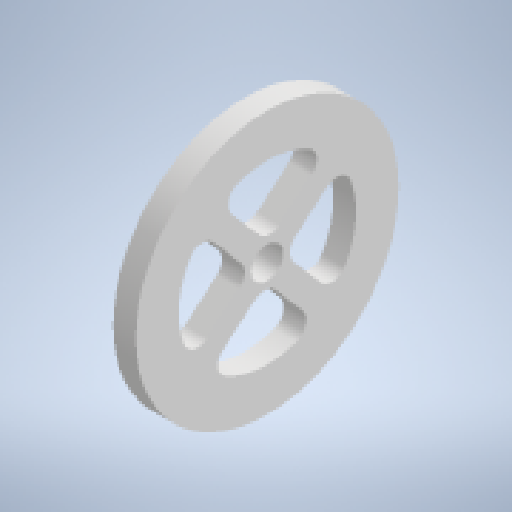
# Autodesk Inventor part: WheelBetter
Saved by Autodesk Inventor 2025.2 (Build 292293000, 293)
## iProperties
Created: 2025-02-03
Part Number: WheelBetter
Material: Generic
Document SubType Name: Modeling
Designer: andre
Density: 1 g/cm^3
Appearance: Default
Author: andre
Autodesk Inventor part; units mm, degrees
ref_plane "YZ Plane" through (0, 0, 0) normal (1, 0, 0) x (0, 1, 0)
ref_plane "XZ Plane" through (0, 0, 0) normal (0, 1, 0) x (-1, 0, 0)
ref_plane "XY Plane" through (0, 0, 0) normal (0, 0, 1) x (1, 0, 0)
sketch "Sketch1" plane through (0, 0, 0) normal (1, 0, 0) x (0, 1, 0)
  arc A0 (23.1835, 24.2674) -> (22.463, 14.9178) centre (33.5654, 18.7649) ccw
  arc A1 (26.4699, 24.6315) -> (23.1835, 24.2674) centre (24.9506, 23.3308) ccw
  line L0 (26.4699, 24.6315) -> (30.0498, 20.4497)
  arc A2 (29.8311, 17.6297) -> (30.0498, 20.4497) centre (28.5305, 19.149) ccw
  line L1 (29.8311, 17.6297) -> (25.6534, 14.0533)
  arc A3 (22.463, 14.9178) -> (25.6534, 14.0533) centre (24.3528, 15.5727) ccw
  arc A4 (28.0629, 8.3829) -> (37.4124, 7.6625) centre (33.5654, 18.7649) ccw
  arc A5 (27.6988, 11.6694) -> (28.0629, 8.3829) centre (28.9995, 10.1501) ccw
  line L2 (27.6988, 11.6694) -> (31.8806, 15.2493)
  arc A6 (34.7006, 15.0306) -> (31.8806, 15.2493) centre (33.1812, 13.73) ccw
  line L3 (34.7006, 15.0306) -> (38.277, 10.8529)
  arc A7 (37.4124, 7.6625) -> (38.277, 10.8529) centre (36.7576, 9.5523) ccw
  arc A8 (43.9473, 13.2623) -> (44.6678, 22.6119) centre (33.5654, 18.7649) ccw
  arc A9 (40.6609, 12.8983) -> (43.9473, 13.2623) centre (42.1802, 14.1989) ccw
  line L4 (40.6609, 12.8983) -> (37.081, 17.0801)
  arc A10 (37.2997, 19.9) -> (37.081, 17.0801) centre (38.6003, 18.3807) ccw
  line L5 (37.2997, 19.9) -> (41.4774, 23.4764)
  arc A11 (44.6678, 22.6119) -> (41.4774, 23.4764) centre (42.778, 21.9571) ccw
  line L6 (32.4303, 22.4992) -> (28.8539, 26.6768)
  arc A12 (29.7184, 29.8673) -> (28.8539, 26.6768) centre (30.3732, 27.9775) ccw
  arc A13 (39.068, 29.1468) -> (29.7184, 29.8673) centre (33.5654, 18.7649) ccw
  arc A14 (39.432, 25.8603) -> (39.068, 29.1468) centre (38.1314, 27.3797) ccw
  line L7 (39.432, 25.8603) -> (35.2502, 22.2805)
  arc A15 (32.4303, 22.4992) -> (35.2502, 22.2805) centre (33.9496, 23.7998) ccw
  circle A16 centre (33.5654, 18.7649) radius 17.5001
  circle A17 centre (33.5654, 18.7649) radius 2.1
  point P0 (0, 0)
  constraints: 32 point on circle, 18 centre point, 16 end point
extrude "Extrusion1" add sketch "Sketch1" along normal blind 3
body "Solid1"
